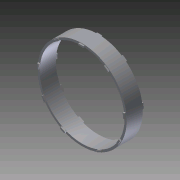
# Autodesk Inventor part: Traction Mount 1764
Saved by Autodesk Inventor 2011 (Build 150239000, 239)
## iProperties
Created: 2009-01-19
Part Number: Traction Mount 1764
Document SubType Name: Modeling
Designer: pmulligan
Density: 1 g/cm^3
Mass: 78.8414 g
Surface Area: 488.462 cm^2
Volume: 78.8414 cm^3
Author: pmulligan
Autodesk Inventor part; units mm, degrees
ref_plane "YZ Plane" through (0, 0, 0) normal (1, 0, 0) x (0, 1, 0)
ref_plane "XZ Plane" through (0, 0, 0) normal (0, 1, 0) x (-1, 0, 0)
ref_plane "XY Plane" through (0, 0, 0) normal (0, 0, 1) x (1, 0, 0)
sketch "Sketch1" plane through (0, 0, 0) normal (0, 0, 1) x (1, 0, 0)
  circle A0 centre (-6.0883, 10.8067) radius 67.0179
  circle A1 centre (-6.0883, 10.8067) radius 70.485
  dimension "d0" = 140.97
  dimension "d1" = 134.0358
  constraints: 2 centre point, 1 coincident
  measures "d0" diameter of A1
  measures "d1" diameter of A0
extrude "Extrusion1" add sketch "Sketch1" along normal blind 25.4
sketch "Sketch2" plane through (-6.0883, 10.8067, 25.4) normal (0, 0, 1) x (1, 0, 0)
  circle A0 centre (0, 0) radius 67.0179 projected
  circle A1 centre (0, 0) radius 70.485 projected
  line L0 (-4.064, 69.6341) -> (4.064, 69.6341)
  line L1 (4.064, 69.6341) -> (4.064, 67.0179)
  line L2 (4.064, 67.0179) -> (-4.064, 67.0179)
  line L3 (-4.064, 67.0179) -> (-4.064, 69.6341)
  line L4 (-43.2695, 54.7099) -> (-36.6114, 59.3719)
  line L5 (-36.6114, 59.3719) -> (-35.1109, 57.2289)
  line L6 (-35.1109, 57.2289) -> (-41.7689, 52.5668)
  line L7 (-41.7689, 52.5668) -> (-43.2695, 54.7099)
  line L8 (36.6114, 59.3719) -> (43.2695, 54.7099)
  line L9 (43.2695, 54.7099) -> (41.7689, 52.5668)
  line L10 (41.7689, 52.5668) -> (35.1109, 57.2289)
  line L11 (35.1109, 57.2289) -> (36.6114, 59.3719)
  line L12 (-69.7233, 2.0205) -> (-69.0149, 10.1175)
  line L13 (-69.0149, 10.1175) -> (-66.4087, 9.8895)
  line L14 (-66.4087, 9.8895) -> (-67.1171, 1.7925)
  line L15 (-67.1171, 1.7925) -> (-69.7233, 2.0205)
  line L16 (-60.0712, -29.9894) -> (-56.0072, -37.0285)
  line L17 (-56.0072, -37.0285) -> (-58.2729, -38.3366)
  line L18 (-58.2729, -38.3366) -> (-62.3369, -31.2975)
  line L19 (-62.3369, -31.2975) -> (-60.0712, -29.9894)
  line L20 (-32.0062, -59.0213) -> (-24.6398, -62.4564)
  line L21 (-24.6398, -62.4564) -> (-25.7454, -64.8274)
  line L22 (-25.7454, -64.8274) -> (-33.1119, -61.3924)
  line L23 (-33.1119, -61.3924) -> (-32.0062, -59.0213)
  line L24 (25.7454, -64.8274) -> (24.6398, -62.4564)
  line L25 (33.1119, -61.3924) -> (25.7454, -64.8274)
  line L26 (32.0062, -59.0213) -> (33.1119, -61.3924)
  line L27 (24.6398, -62.4564) -> (32.0062, -59.0213)
  line L28 (69.0149, 10.1175) -> (69.7233, 2.0205)
  line L29 (69.7233, 2.0205) -> (67.1171, 1.7925)
  line L30 (67.1171, 1.7925) -> (66.4087, 9.8895)
  line L31 (66.4087, 9.8895) -> (69.0149, 10.1175)
  line L32 (62.3369, -31.2975) -> (58.2729, -38.3366)
  line L33 (58.2729, -38.3366) -> (56.0072, -37.0285)
  line L34 (56.0072, -37.0285) -> (60.0712, -29.9894)
  line L35 (60.0712, -29.9894) -> (62.3369, -31.2975)
  line L36 (33.1119, -61.3924) -> (25.7454, -64.8274)
  line L37 (25.7454, -64.8274) -> (24.6398, -62.4564)
  line L38 (24.6398, -62.4564) -> (32.0062, -59.0213)
  line L39 (32.0062, -59.0213) -> (33.1119, -61.3924)
  dimension "d4" = 2.6162
  dimension "d5" = 8.128
  dimension "d8" = 35
  dimension "d12" = 35
  dimension "d16" = 50
  dimension "d20" = 70
  dimension "d24" = 50
  dimension "d28" = 50
  dimension "d32" = 70
  constraints: 80 end point, 2 parallel, 1 horizontal, 1 perpendicular, 79 other
  measures "d4" distance of L2.end L0.start
  measures "d5" distance of L0.start L0.end
extrude "Extrusion2" add sketch "Sketch2" along normal blind 2.2352 contours L34 L35 L32 L33 | L27 L26 L25 L24 | L20 L21 L22 L23 | L16 L17 L18 L19 | L14 L15 L12 L13 | L6 L7 L4 L5 | L2 L3 L0 L1 | L10 L11 L8 L9 | L30 L31 L28 L29
sketch "Sketch3" plane through (-6.0883, 10.8067, 0) normal (0, 0, -1) x (-1, 0, 0)
  line L0 (-4.064, 67.0179) -> (4.064, 67.0179)
  line L1 (4.064, 67.0179) -> (4.064, 69.6341)
  line L2 (4.064, 69.6341) -> (-4.064, 69.6341)
  line L3 (-4.064, 69.6341) -> (-4.064, 67.0179)
  line L4 (-35.1109, 57.2289) -> (-36.6114, 59.3719)
  line L5 (-36.6114, 59.3719) -> (-43.2695, 54.7099)
  line L6 (-41.7689, 52.5668) -> (-35.1109, 57.2289)
  line L7 (-43.2695, 54.7099) -> (-41.7689, 52.5668)
  line L8 (-69.7233, 2.0205) -> (-67.1171, 1.7925)
  line L9 (-69.0149, 10.1175) -> (-69.7233, 2.0205)
  line L10 (-66.4087, 9.8895) -> (-69.0149, 10.1175)
  line L11 (-67.1171, 1.7925) -> (-66.4087, 9.8895)
  line L12 (-60.0712, -29.9894) -> (-62.3369, -31.2975)
  line L13 (-56.0072, -37.0285) -> (-60.0712, -29.9894)
  line L14 (-58.2729, -38.3366) -> (-56.0072, -37.0285)
  line L15 (-62.3369, -31.2975) -> (-58.2729, -38.3366)
  line L16 (36.6114, 59.3719) -> (35.1109, 57.2289)
  line L17 (43.2695, 54.7099) -> (36.6114, 59.3719)
  line L18 (41.7689, 52.5668) -> (43.2695, 54.7099)
  line L19 (35.1109, 57.2289) -> (41.7689, 52.5668)
  line L20 (-32.0062, -59.0213) -> (-33.1119, -61.3924)
  line L21 (-24.6398, -62.4564) -> (-32.0062, -59.0213)
  line L22 (-25.7454, -64.8274) -> (-24.6398, -62.4564)
  line L23 (-33.1119, -61.3924) -> (-25.7454, -64.8274)
  line L24 (32.0062, -59.0213) -> (24.6398, -62.4564)
  line L25 (33.1119, -61.3924) -> (32.0062, -59.0213)
  line L26 (25.7454, -64.8274) -> (33.1119, -61.3924)
  line L27 (24.6398, -62.4564) -> (25.7454, -64.8274)
  line L28 (60.0712, -29.9894) -> (56.0072, -37.0285)
  line L29 (62.3369, -31.2975) -> (60.0712, -29.9894)
  line L30 (58.2729, -38.3366) -> (62.3369, -31.2975)
  line L31 (56.0072, -37.0285) -> (58.2729, -38.3366)
  line L32 (69.0149, 10.1175) -> (66.4087, 9.8895)
  line L33 (69.7233, 2.0205) -> (69.0149, 10.1175)
  line L34 (67.1171, 1.7925) -> (69.7233, 2.0205)
  line L35 (66.4087, 9.8895) -> (67.1171, 1.7925)
extrude "Extrusion3" add sketch "Sketch3" along normal blind 2.2352
body "Solid1"
